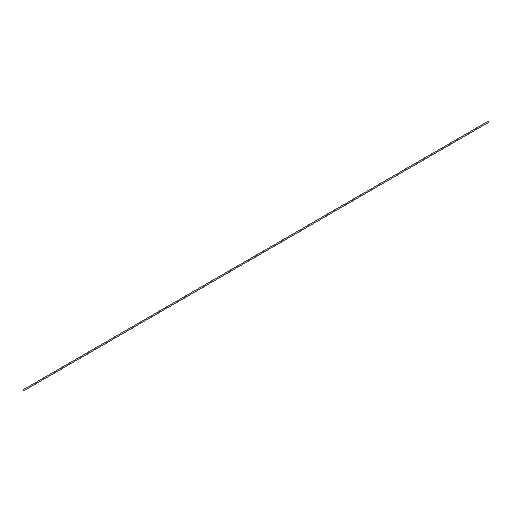
# Autodesk Inventor part: model
Saved by Autodesk Inventor 2025 (Build 290162000, 162)
## iProperties
Created: 2024-05-18
Part Number: model
Material: Generic
Document SubType Name: Modeling
Designer: tinas
Density: 1 g/cm^3
Appearance: Default
Author: tinas
Autodesk Inventor part; units mm, degrees
ref_plane "YZ Plane" through (0, 0, 0) normal (1, 0, 0) x (0, 1, 0)
ref_plane "XZ Plane" through (0, 0, 0) normal (0, 1, 0) x (-1, 0, 0)
ref_plane "XY Plane" through (0, 0, 0) normal (0, 0, 1) x (1, 0, 0)
sketch "Sketch1" plane through (0, 0, 0) normal (0, 0, 1) x (1, 0, 0)
  line L0 (-50, 1134) -> (50, 1134)
  line L1 (50, 1134) -> (50, -1134)
  line L2 (50, -1134) -> (-50, -1134)
  line L3 (-50, -1134) -> (-50, 1134)
  line L4 (-70, 0) -> (70, 0) projected
  line L5 (0, -1587.6) -> (0, 1587.6) projected
  point P0 (0, 0)
  dimension "d0" = 2268
  dimension "d1" = 100
  constraints: 8 end point, 2 parallel, 1 horizontal, 1 perpendicular, 2 other
  measures "d0" distance of L0.end L1.end
  measures "d1" distance of L0.start L0.end
extrude "Extrusion1" add sketch "Sketch1" along normal mid plane 879000
body "Solid1"
